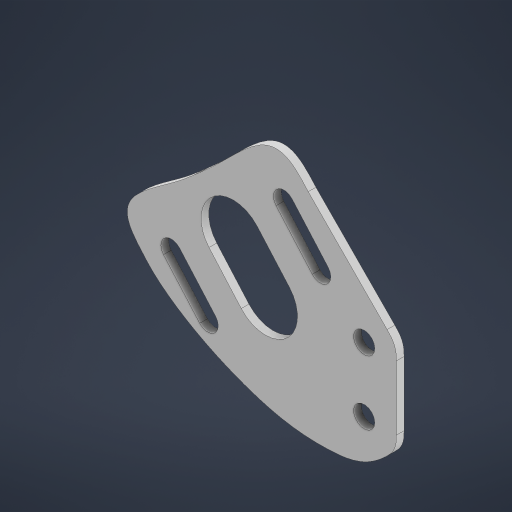
# Autodesk Inventor part: third-stage
Saved by Autodesk Inventor 2023 (Build 270158000, 158)
## iProperties
Created: 2023-03-29
Part Number: third-stage
Material: Generic
Document SubType Name: Modeling
Designer: Liam
Density: 1 g/cm^3
Appearance: Default
Author: Liam
Autodesk Inventor part; units mm, degrees
ref_plane "YZ Plane" through (0, 0, 0) normal (1, 0, 0) x (0, 1, 0)
ref_plane "XZ Plane" through (0, 0, 0) normal (0, 1, 0) x (-1, 0, 0)
ref_plane "XY Plane" through (0, 0, 0) normal (0, 0, 1) x (1, 0, 0)
sketch "Sketch1" plane through (0, 0, 0) normal (0, 0, 1) x (1, 0, 0)
  circle A0 centre (-71.5229, 62.251) radius 6.35
  line L0 (-85.2902, 52.3318) -> (-78.1339, 44.1713)
  line L1 (-74.9829, 46.9345) -> (-82.1391, 55.0951)
  arc A1 (-78.1339, 44.1713) -> (-74.9829, 46.9345) centre (-76.5584, 45.5529) ccw
  arc A2 (-82.1391, 55.0951) -> (-85.2902, 52.3318) centre (-83.7146, 53.7134) ccw
  line L2 (-63.042, 71.842) -> (-55.8858, 63.6815)
  line L3 (-52.7347, 66.4447) -> (-59.891, 74.6052)
  arc A3 (-55.8858, 63.6815) -> (-52.7347, 66.4447) centre (-54.3102, 65.0631) ccw
  arc A4 (-59.891, 74.6052) -> (-63.042, 71.842) centre (-61.4665, 73.2236) ccw
  line L4 (-61.4665, 73.2236) -> (-83.7146, 53.7134)
  circle A5 centre (-45.6184, 44.45) radius 2.0955
  circle A6 centre (-45.6184, 57.15) radius 2.0955
  line L5 (-38.1, 63.5) -> (-38.1, 38.1) projected
  line L6 (-71.5229, 62.251) -> (-78.2217, 69.8899)
  line L7 (-61.4665, 73.2236) -> (-56.6922, 77.4103)
  line L8 (-83.7146, 53.7134) -> (-88.4889, 49.5267)
  line L9 (-78.2217, 69.8899) -> (-79.1765, 69.0525)
  line L10 (-88.4889, 49.5267) -> (-89.3263, 50.4816)
  spline S0 degree 4 poles (-89.3263, 50.4816) (-91.643, 53.1234) (-96.2764, 58.4071) (-85.3251, 63.6606) (-81.226, 67.2552) (-79.1765, 69.0525) knots 0 0 0 0 0 0.5 1 1 1 1 1
  line L11 (-56.6922, 77.4103) -> (-57.5295, 78.3652)
  line L12 (-78.2217, 69.8899) -> (-77.2668, 70.7272)
  spline S1 degree 4 poles (-78.2217, 69.8899) (-76.0004, 71.8378) (-71.5579, 75.7336) (-64.0941, 85.8511) (-59.1595, 80.2239) (-56.6922, 77.4103) knots 0 0 0 0 0 0.5 1 1 1 1 1
  line L13 (-56.6922, 77.4103) -> (-41.0988, 61.6105)
  line L14 (-88.4889, 49.5267) -> (-86.4935, 47.2513) construction
  line L15 (-86.4935, 47.2513) -> (-79.1765, 41.658) construction
  line L16 (-79.1765, 41.658) -> (-65.6397, 36.2801) construction
  line L17 (-65.6397, 36.2801) -> (-57.5295, 35.1145) construction
  line L18 (-57.5295, 35.1145) -> (-50.9347, 35.1145) construction
  line L19 (-50.9347, 35.1145) -> (-45.158, 36.0858) construction
  line L20 (-45.158, 36.0858) -> (-41.2186, 39.8714) construction
  spline S2 degree 4 poles (-88.4889, 49.5267) (-86.4935, 47.2513) (-79.1765, 41.658) (-65.6397, 36.2801) (-57.5295, 35.1145) (-50.9347, 35.1145) (-45.158, 36.0858) (-41.2186, 39.8714) knots 1 1 1 1 1 2 3 4 5 5 5 5 5
  line L21 (-39.2684, 44.45) -> (-39.2684, 57.15)
  spline S3 degree 4 poles (-39.2684, 57.15) (-39.2684, 57.7752) (-39.2684, 59.0257) (-39.7812, 60.2755) (-40.6596, 61.1655) (-41.0988, 61.6105) knots 0 0 0 0 0 0.5 1 1 1 1 1
  spline S4 degree 4 poles (-39.2684, 44.45) (-39.2684, 43.803) (-39.2684, 42.5091) (-39.8191, 41.2162) (-40.7521, 40.3196) (-41.2186, 39.8714) knots 0 0 0 0 0 0.5 1 1 1 1 1
  line L22 (-76.2972, 58.0643) -> (-69.9264, 50.7994)
  line L23 (-66.7486, 66.4377) -> (-60.3778, 59.1729)
  arc A7 (-69.9264, 50.7994) -> (-60.3778, 59.1729) centre (-65.1521, 54.9861) ccw
  point P0 (0, 0)
  point P1 (-79.2989, 51.8562)
  dimension "d0" = 12.7
  dimension "d4" = 180
  dimension "d5" = 4.191
  dimension "d7" = 180
  dimension "d8" = 4.191
  dimension "d12" = 29.591
  dimension "d14" = 6.35
  dimension "d15" = 6.35
  dimension "d18" = 1.27
  dimension "d19" = 10.16
  dimension "d20" = 1.27
  dimension "d21" = 1.27
  dimension "d22" = 1.27
  dimension "d23" = 4.191
  dimension "d24" = 4.191
  constraints: 32 end point, 12 point on circle, 8 centre point, 7 tangent, 6 parallel, 5 perpendicular, 2 collinear, 2 point on line, 2 vertical, 1 horizontal, 22 other
  measures "d0" diameter of A0
  measures "d5" distance between parallel lines of L1 L0
  measures "d8" distance between parallel lines of L3 L2
  measures "d12" distance of L4.start L4.end
  measures "d14" distance of L4.start L7.end
  measures "d15" distance of L4.end L8.end
  measures "d18" distance of L6.end L9.end
  measures "d19" distance of L6.start L6.end
  measures "d20" distance of L8.end L10.end
  measures "d21" distance of L7.end L11.end
  measures "d22" distance of L6.end L12.end
  measures "d23" diameter of A5
  measures "d24" diameter of A6
extrude "Extrusion2" add sketch "Sketch1" along normal blind 1.524 contours A0 L4 L2 A3 L3 L7 L13 S3 L21 S4 S2 L8 L0 A1 L1 L22 A7 L23 | A0 L6 S1 L7 A4 L4 | L4 A2 L8 L10 S0 L9 L6 A0
body "Solid2"
